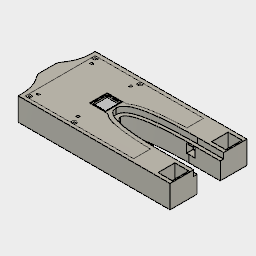
Plattan från fusion (Autodesk Fusion 360 design; units mm, degrees)
Autodesk Fusion 360 part; units mm, degrees
note: some values were not read from the file. Set by a fixed rule: which face or edge a step refers to.
(part 1 of 2)
sketch "Sketch1" plane through (0, 0, 0) normal (0, 1, 0) x (1, 0, 0)
  line L0 (220, -110) -> (0, -110)
  line L1 (0, -110) -> (0, 0)
  line L2 (220, -71.2097) -> (220, -110)
  line L3 (0, 0) -> (220, 0)
  line L4 (5, -5) -> (215, -5)
  line L5 (215, -5) -> (215, -33.4693)
  line L6 (180.0334, -33.4693) -> (215, -33.4693)
  spline S0 degree 3 poles (180.0334, -33.4693) (180.0317, -33.4693) (180.03, -33.4693) (180.0283, -33.4693) (159.0681, -33.512) (139.654, -34.3205) (124.0136, -36.2172) (115.4073, -37.2609) (107.9508, -38.6227) (101.8781, -40.4563) (97.9385, -41.6458) (94.574, -43.0141) (91.7704, -44.8227) (89.9877, -45.9727) (88.4083, -47.3156) (87.1811, -49.0361) (86.1319, -50.5071) (85.3713, -52.2924) (85.1516, -54.1891) (85.1143, -54.5109) (85.0919, -54.8348) (85.0844, -55.1587) (85.0841, -55.173) (85.0838, -55.1872) (85.0834, -55.2015) knots 0.561232 0.561232 0.561232 0.561232 0.561247 0.561247 0.561247 0.747063 0.747063 0.747063 0.849312 0.849312 0.849312 0.915644 0.915644 0.915644 0.957822 0.957822 0.957822 0.993882 0.993882 0.993882 1 1 1 1.000508 1.000508 1.000508 1.000508
  spline S1 degree 3 poles (85.0834, -55.2015) (85.0833, -55.2157) (85.0832, -55.23) (85.0832, -55.2442) (85.0717, -57.1054) (85.5912, -58.9664) (86.472, -60.5273) (87.5859, -62.5014) (89.1837, -64.0174) (90.9945, -65.2727) (93.6691, -67.1266) (96.8885, -68.4839) (100.6688, -69.6551) (106.9846, -71.6118) (114.9032, -72.9866) (124.1531, -73.9888) (139.7696, -75.6808) (159.1421, -76.258) (180.0619, -76.065) knots -0.00051 -0.00051 -0.00051 -0.00051 0 0 0 0.035213 0.035213 0.035213 0.079749 0.079749 0.079749 0.145527 0.145527 0.145527 0.255424 0.255424 0.255424 0.440962 0.440962 0.440962 0.440962
  line L7 (180.0619, -76.065) -> (215, -76.065)
  line L8 (215, -76.065) -> (215, -105)
  line L9 (215, -105) -> (5, -105)
  line L10 (5, -105) -> (5, -5)
  line L11 (220, -71.2097) -> (220, -76.065)
  line L12 (215, -92) -> (205, -92)
  line L13 (215, -18) -> (205, -18)
  circle A0 centre (205, -92) radius 2.7
  circle A1 centre (205, -18) radius 2.7
  circle A2 centre (205, -92) radius 5.25
  circle A3 centre (205, -18) radius 5.25
  line L14 (180.085, -81.065) -> (215, -81.065)
  spline S2 degree 3 poles (80.0838, -55.128) (80.0836, -55.1565) (80.0834, -55.1851) (80.0833, -55.2136) (80.0693, -57.4847) (80.5939, -59.807) (81.5103, -61.7976) (82.5316, -64.0162) (83.9716, -65.8142) (85.5066, -67.2576) (87.6935, -69.3141) (90.0877, -70.738) (92.6384, -71.9379) (96.4174, -73.7157) (100.6123, -74.9881) (105.3471, -76.0639) (113.1343, -77.8331) (122.3837, -79.0075) (132.8521, -79.8035) (146.8378, -80.8669) (162.9619, -81.2225) (180.085, -81.065) knots -0.00102 -0.00102 -0.00102 -0.00102 0 0 0 0.029213 0.029213 0.029213 0.061771 0.061771 0.061771 0.108156 0.108156 0.108156 0.176878 0.176878 0.176878 0.2899 0.2899 0.2899 0.440894 0.440894 0.440894 0.440894
  spline S3 degree 3 poles (180.0283, -28.4693) (180.0249, -28.4693) (180.0215, -28.4693) (180.0181, -28.4693) (162.2889, -28.5054) (145.6262, -29.0859) (131.2931, -30.4153) (122.4806, -31.2327) (114.5551, -32.326) (107.6808, -33.8168) (102.9997, -34.8321) (98.8082, -36.0189) (95.0386, -37.5637) (92.2561, -38.7039) (89.687, -40.0255) (87.3028, -41.8568) (85.5074, -43.2358) (83.7899, -44.9342) (82.4288, -47.164) (81.3112, -48.9949) (80.4774, -51.2077) (80.1955, -53.5241) (80.134, -54.0286) (80.0975, -54.5363) (80.0858, -55.0425) (80.0851, -55.071) (80.0844, -55.0995) (80.0838, -55.128) knots 0.561217 0.561217 0.561217 0.561217 0.561247 0.561247 0.561247 0.717499 0.717499 0.717499 0.813569 0.813569 0.813569 0.878987 0.878987 0.878987 0.927274 0.927274 0.927274 0.963637 0.963637 0.963637 0.993496 0.993496 0.993496 1 1 1 1.001016 1.001016 1.001016 1.001016
  line L15 (180.0283, -28.4693) -> (215, -28.4693)
  line L16 (205, -92) -> (195, -92)
  line L17 (195, -92) -> (195, -105)
  line L18 (195, -92) -> (195, -81.065)
  line L19 (195, -105) -> (160, -105)
  line L20 (160, -105) -> (160, -80.9937)
  line L21 (160, -28.7673) -> (160, -5)
  line L22 (160, -5) -> (195, -5)
  line L23 (195, -5) -> (195, -28.4693)
  line L24 (220, -33.4693) -> (220, -33.4693)
  line L25 (220, -76.065) -> (220.0001, -76.065)
  line L26 (160, -28.7673) -> (160, -33.7693)
  line L27 (195, -28.4693) -> (195, -33.4693)
  line L28 (195, -81.065) -> (195, -76.065)
  line L29 (160, -80.9937) -> (160, -75.9932)
  line L30 (215, -107.6) -> (2.4, -107.6)
  line L31 (2.4, -107.6) -> (2.4, -2.4)
  line L32 (2.4, -2.4) -> (215, -2.4)
  line L33 (215, -5) -> (215, -2.4)
  line L34 (215, -105) -> (215, -107.6)
  line L35 (80.0839, -55) -> (80.0868, -55)
  line L36 (80.0868, -55) -> (80.0868, -65)
  line L37 (80.0868, -65) -> (62.0868, -65)
  line L38 (62.0868, -65) -> (62.0868, -45)
  line L39 (62.0868, -45) -> (80.0868, -45)
  line L40 (80.0868, -45) -> (80.0868, -65)
  line L41 (82.0868, -67) -> (60.0868, -67)
  line L42 (60.0868, -67) -> (60.0868, -43)
  line L43 (60.0868, -43) -> (82.0868, -43)
  line L44 (82.0868, -43) -> (82.0868, -67)
  line L45 (80.8868, -65.8) -> (61.2868, -65.8)
  line L46 (61.2868, -65.8) -> (61.2868, -44.2)
  line L47 (61.2868, -44.2) -> (80.8868, -44.2)
  line L48 (80.8868, -44.2) -> (80.8868, -65.8)
  line L49 (215, -33.4693) -> (220, -33.4693)
  line L50 (215, -76.065) -> (220.0001, -76.065)
  spline S4 degree 3 poles (172.3167, -38.2821) (127.2999, -38.721) (91.6663, -43.1669) (91.3547, -54.7171) knots 0.588488 0.588488 0.588488 0.588488 1 1 1 1
  line L51 (172.3978, -71.2493) -> (220, -71.2097)
  line L52 (172.3167, -38.2821) -> (220, -38.2821)
  spline S5 degree 3 poles (91.3547, -54.7171) (91.1824, -66.3112) (127.02, -70.7779) (172.3978, -71.2493) knots 0 0 0 0 0.414646 0.414646 0.414646 0.414646
  line L53 (220, -76.065) -> (220, -71.2097)
  line L54 (220, -38.2821) -> (220, 0)
  line L55 (80.0868, -67.8) -> (59.2868, -67.8)
  line L56 (59.2868, -67.8) -> (59.2868, -42.2)
  line L57 (59.2868, -42.2) -> (80.0868, -42.2)
  line L58 (80.0868, -42.2) -> (86.8661, -42.2)
  line L59 (80.0868, -67.8) -> (86.1046, -67.8)
  dimension "d1" = 110
  dimension "d2" = 220
  dimension "d33" = 5.4
  dimension "d34" = 5.4
  dimension "d35" = 10.5
  dimension "d36" = 10.5
  dimension "d38" = 10
  dimension "d43" = 35
  dimension "d44" = 35
  dimension "d47" = 5
  dimension "d65" = 10
  dimension "d66" = 18
  dimension "d67" = 20
  dimension "d68" = 2
  dimension "d69" = 0.8
  dimension "d447" = 2.8
  measures "d1" distance of L1.end L0.end
  measures "d2" distance of L1.end L3.end
  measures "d33" diameter of A0
  measures "d34" diameter of A1
  measures "d35" diameter of A2
  measures "d36" diameter of A3
  measures "d38" distance of L12.end L16.end
  measures "d43" distance of L17.end L19.end
  measures "d44" distance of L21.end L22.end
  measures "d47" distance of L5.end L24.start
  measures "d65" distance of L35.end L36.end
  measures "d66" distance of L36.end L37.end
  measures "d67" distance of L36.end L39.end
extrude "Extrude51" add sketch "Sketch1" against normal blind 3 contours S2 S3 L41 L42 L43 L44 L55 L56 L57 L58 L59 | S2 S3 L41 L42 L43 L44 L45 L46 L47 L48 | S2 S3 L36 L37 L38 L39 L40 L45 L46 L47 L48 makes body 1
extrude "Extrude17" add sketch "Sketch1" along normal blind 0.7 separate body contours L0 L1 L2 L3 L5 L8 L30 L31 L32 L33 L34 L49 L50 L54 | L2 L6 S0 S1 L7 L11 L49 L50 S4 L51 L52 S5 L53 L54 | L7 L8 L14 L28 | S1 L7 L14 S2 L28 L29 | L9 L14 S2 L17 L18 L19 L20 | L5 L6 L15 L27 | S0 S1 S2 S3 L26 L29 L44 | L4 L9 L10 L19 L22 L30 L31 L32 L33 L34 | L6 S0 S3 L15 L26 L27 | L4 L9 L10 S2 S3 L20 L21 L55 L56 L57 L58 L59 | L4 S3 L15 L21 L22 L23 | S2 S3 L41 L42 L43 L44 L55 L56 L57 L58 L59 | S2 S3 L41 L42 L43 L44 L45 L46 L47 L48 | S2 S3 L44 L48 | S2 S3 L36 L37 L38 L39 L40 L45 L46 L47 L48 | S2 S3 L36 L40 L48 | S2 S3 L36 L37 L38 L39 L40 | S2 S3 L36 L40 makes body 2
extrude "Extrude15" add sketch "Sketch1" against normal blind 32 contours L0 L1 L2 L3 L5 L8 L30 L31 L32 L33 L34 L49 L50 L54 | L2 L6 S0 S1 L7 L11 L49 L50 S4 L51 L52 S5 L53 L54 bodies 2
extrude "Extrude18" add sketch "Sketch1" against normal blind 28 contours L7 L8 L14 L28 | S1 L7 L14 S2 L28 L29 | L9 L14 S2 L17 L18 L19 L20 | L5 L6 L15 L27 | S0 S1 S2 S3 L26 L29 L44 | L4 L9 L10 L19 L22 L30 L31 L32 L33 L34 | L6 S0 S3 L15 L26 L27 | L4 S3 L15 L21 L22 L23 | S2 S3 L44 L48 | S2 S3 L36 L40 L48 | S2 S3 L36 L40 bodies 2
extrude "Extrude19" cut sketch "Sketch1" along normal through all contours S2 S3 L36 L37 L38 L39 L40 bodies 2
sketch "Sketch7" plane through (0, 0, 0) normal (0, 0, -1) x (-1, 0, 0)
  line L0 (0, -32) -> (0, 0.7)
  line L1 (0, 0.7) -> (-220, 0.7)
  line L2 (-220, -32) -> (0, -32)
  line L3 (-220, 0.7) -> (-190, 0.7156)
  line L4 (-190, 0.7156) -> (-190, -32)
  line L5 (-181, -9.5928) -> (-180.9904, -9.5928)
  line L6 (-181, -9.5928) -> (-180.9904, -21.5928)
  line L7 (-180.9904, -21.5928) -> (-168.9904, -21.5928)
  line L8 (-168.9904, -21.5928) -> (-168.9904, -9.5928)
  line L9 (-168.9904, -9.5928) -> (-180.9904, -9.5928)
  line L10 (-180.9904, -9.5928) -> (-180.9904, -21.5928)
  line L11 (-190, -32) -> (-160, -32)
  line L12 (-160, -32) -> (-160, 0.7)
  line L13 (-220, 0.7) -> (-220, -32)
  dimension "d77" = 30
  dimension "d127" = 12
  dimension "d128" = 12
  dimension "d129" = 12
  dimension "d130" = 30
  measures "d77" distance of L1.end L3.end
  measures "d127" distance of L5.start L6.end
  measures "d128" distance of L6.end L5.end
  measures "d129" distance of L6.end L7.end
  measures "d130" distance of L4.end L11.end
extrude "Extrude25" cut sketch "Sketch7" against normal blind 10 from surface at -29 contours L7 L8 L9 L10 bodies 2
sketch "Sketch8" plane through (0, 0.7, 0) normal (0, 1, 0) x (-1, 0, 0)
  line L0 (-195, 105) -> (-195, 81.065)
  line L1 (-195, 81.065) -> (-215, 81.065)
  line L2 (-215, 81.065) -> (-215, 105)
  line L3 (-215, 105) -> (-195, 105)
  line L4 (-195, 5) -> (-215, 5)
  line L5 (-215, 5) -> (-215, 28.4693)
  line L6 (-215, 28.4693) -> (-195, 28.4693)
  line L7 (-195, 28.4693) -> (-195, 5)
  line L8 (-220, 0) -> (0, 0)
  line L9 (0, 0) -> (0, 110)
  line L10 (0, 110) -> (-220, 110)
  line L11 (-220, 110) -> (-220, 71.2097)
  line L12 (-220, 76.065) -> (-180.0619, 76.065)
  spline S0 degree 3 poles (-180.0619, 76.065) (-159.1795, 76.2576) (-139.8387, 75.6828) (-124.2368, 73.9979) (-115.6615, 73.0718) (-108.2229, 71.8213) (-102.1502, 70.0947) (-98.213, 68.9753) (-94.844, 67.6751) (-92.0221, 65.9426) (-90.1417, 64.7881) (-88.4752, 63.4272) (-87.1878, 61.6436) (-86.1381, 60.1892) (-85.3752, 58.4147) (-85.1541, 56.5302) (-85.104, 56.1036) (-85.0805, 55.6734) (-85.0832, 55.2442) (-85.0832, 55.23) (-85.0833, 55.2157) (-85.0834, 55.2015) knots -0.440962 -0.440962 -0.440962 -0.440962 -0.255755 -0.255755 -0.255755 -0.153959 -0.153959 -0.153959 -0.087961 -0.087961 -0.087961 -0.04398 -0.04398 -0.04398 -0.008119 -0.008119 -0.008119 0 0 0 0.00051 0.00051 0.00051 0.00051
  spline S1 degree 3 poles (-85.0834, 55.2015) (-85.0838, 55.1872) (-85.0841, 55.173) (-85.0844, 55.1587) (-85.1283, 53.2729) (-85.7115, 51.4171) (-86.6378, 49.8664) (-87.8395, 47.8546) (-89.5287, 46.3185) (-91.4514, 45.0322) (-94.4377, 43.0345) (-98.0815, 41.5688) (-102.3978, 40.3015) (-109.8672, 38.1085) (-119.3843, 36.5903) (-130.4817, 35.5147) (-144.8663, 34.1205) (-161.8701, 33.5063) (-180.0283, 33.4693) (-180.03, 33.4693) (-180.0317, 33.4693) (-180.0334, 33.4693) knots -1.000508 -1.000508 -1.000508 -1.000508 -1 -1 -1 -0.964386 -0.964386 -0.964386 -0.918178 -0.918178 -0.918178 -0.846413 -0.846413 -0.846413 -0.722224 -0.722224 -0.722224 -0.561247 -0.561247 -0.561247 -0.561232 -0.561232 -0.561232 -0.561232
  line L13 (-180.0334, 33.4693) -> (-220, 33.4693)
  line L14 (-172.3167, 38.2821) -> (-220, 38.2821)
  line L15 (-220, 38.2821) -> (-220, 0)
  line L16 (-220, 71.2097) -> (-172.3978, 71.2493)
  spline S2 degree 3 poles (-172.3978, 71.2493) (-127.02, 70.7779) (-91.1824, 66.3112) (-91.3547, 54.7171) knots -0.414646 -0.414646 -0.414646 -0.414646 0 0 0 0
  spline S3 degree 3 poles (-91.3547, 54.7171) (-91.6663, 43.1669) (-127.2999, 38.721) (-172.3167, 38.2821) knots -1 -1 -1 -1 -0.588488 -0.588488 -0.588488 -0.588488
  line L17 (-80.0868, 65) -> (-62.0868, 65)
  line L18 (-62.0868, 65) -> (-62.0868, 45)
  line L19 (-62.0868, 45) -> (-80.0868, 45)
  line L20 (-80.0868, 45) -> (-80.0868, 55)
  spline S4 degree 3 poles (-80.0868, 55) (-80.0864, 55.0142) (-80.0861, 55.0283) (-80.0858, 55.0425) (-80.0851, 55.071) (-80.0844, 55.0995) (-80.0838, 55.128) knots 0.999818 0.999818 0.999818 0.999818 1 1 1 1.001016 1.001016 1.001016 1.001016
  spline S5 degree 3 poles (-80.0838, 55.128) (-80.0836, 55.1565) (-80.0834, 55.1851) (-80.0833, 55.2136) (-80.0824, 55.354) (-80.0836, 55.4946) (-80.0868, 55.6354) knots -0.00102 -0.00102 -0.00102 -0.00102 0 0 0 0.001806 0.001806 0.001806 0.001806
  line L21 (-80.0868, 55.6354) -> (-80.0868, 65)
extrude "Extrude22" cut sketch "Sketch8" against normal blind 8 contours L11 L12 S0 S1 L13 L14 L15 L16 S2 S3 bodies 2
sketch "Sketch9" plane through (0, 0, 110) normal (0, 0, 1) x (1, 0, 0)
  line L0 (220, -32) -> (220, 0.7)
  line L1 (220, 0.7) -> (0, 0.7)
  line L2 (0, 0.7) -> (0, -32)
  line L3 (0, -32) -> (220, -32)
  line L4 (176.1, -28.0515) -> (176.1, -26.85)
  line L5 (173.9, -26.85) -> (173.9, -28.0515)
  arc A0 (176.1, -26.85) -> (173.9, -26.85) centre (175, -26.85) ccw
  line L6 (186.25, -16.7) -> (187.4515, -16.7)
  arc A1 (186.25, -14.5) -> (186.25, -16.7) centre (186.25, -15.6) ccw
  line L7 (187.4515, -14.5) -> (186.25, -14.5)
  line L8 (173.9, -3.1485) -> (173.9, -4.35)
  line L9 (176.1, -4.35) -> (176.1, -3.1485)
  arc A2 (173.9, -4.35) -> (176.1, -4.35) centre (175, -4.35) ccw
  line L10 (186.25, -16.7) -> (187.4515, -16.7)
  arc A3 (186.25, -14.5) -> (186.25, -16.7) centre (186.25, -15.6) ccw
  line L11 (173.9, -3.1485) -> (173.9, -4.35)
  line L12 (187.4515, -14.5) -> (186.25, -14.5)
  arc A4 (173.9, -4.35) -> (176.1, -4.35) centre (175, -4.35) ccw
  line L13 (158, -15.6) -> (158, -11.1)
  line L14 (176.1, -28.0515) -> (176.1, -26.85)
  line L15 (176.1, -4.35) -> (176.1, -3.1485)
  line L16 (173.9, -26.85) -> (173.9, -28.0515)
  arc A5 (176.1, -26.85) -> (173.9, -26.85) centre (175, -26.85) ccw
  arc A6 (176.1, -26.85) -> (173.9, -26.85) centre (175, -26.85) ccw
  arc A7 (173.9, -4.35) -> (176.1, -4.35) centre (175, -4.35) ccw
  line L17 (176.1, -4.35) -> (176.1, -3.1485)
  arc A8 (176.1, -26.85) -> (173.9, -26.85) centre (175, -26.85) ccw
  arc A9 (173.9, -4.35) -> (176.1, -4.35) centre (175, -4.35) ccw
  line L18 (176.1, -28.0515) -> (176.1, -26.85)
  line L19 (173.9, -26.85) -> (173.9, -28.0515)
  line L20 (186.25, -16.7) -> (187.4515, -16.7)
  line L21 (158, -15.6) -> (158, -20.1)
  line L22 (173.9, -3.1485) -> (173.9, -4.35)
  line L23 (176.1, -28.0515) -> (176.1, -26.85)
  line L24 (176.1, -4.35) -> (176.1, -3.1485)
  line L25 (173.9, -3.1485) -> (173.9, -4.35)
  line L26 (173.9, -26.85) -> (173.9, -28.0515)
  line L27 (187.4515, -14.5) -> (186.25, -14.5)
  arc A10 (186.25, -14.5) -> (186.25, -16.7) centre (186.25, -15.6) ccw
  line L28 (186.25, -16.7) -> (187.4515, -16.7)
  arc A11 (186.25, -14.5) -> (186.25, -16.7) centre (186.25, -15.6) ccw
  line L29 (187.4515, -14.5) -> (186.25, -14.5)
  arc A12 (173.9, -4.35) -> (176.1, -4.35) centre (175, -4.35) ccw
  arc A13 (173.9, -4.35) -> (176.1, -4.35) centre (175, -4.35) ccw
  arc A14 (173.9, -4.35) -> (176.1, -4.35) centre (175, -4.35) ccw
  arc A15 (173.9, -4.35) -> (176.1, -4.35) centre (175, -4.35) ccw
  line L30 (176.1, -4.35) -> (176.1, -3.1485)
  line L31 (173.9, -3.1485) -> (173.9, -4.35)
  line L32 (176.1, -4.35) -> (176.1, -3.1485)
  line L33 (173.9, -3.1485) -> (173.9, -4.35)
  line L34 (173.9, -3.1485) -> (173.9, -4.35)
  line L35 (176.1, -4.35) -> (176.1, -3.1485)
  line L36 (173.9, -3.1485) -> (173.9, -4.35)
  line L37 (158, -11.1) -> (164.3229, -9.1)
  line L38 (158, -20.1) -> (158, -30)
  arc A16 (176.1, -26.85) -> (173.9, -26.85) centre (175, -26.85) ccw
  line L39 (173.9, -26.85) -> (173.9, -28.0515)
  line L40 (186.25, -16.7) -> (187.4515, -16.7)
  line L41 (187.4515, -14.5) -> (186.25, -14.5)
  line L42 (187.4515, -14.5) -> (186.25, -14.5)
  line L43 (186.25, -16.7) -> (187.4515, -16.7)
  line L44 (187.4515, -14.5) -> (186.25, -14.5)
  arc A17 (186.25, -14.5) -> (186.25, -16.7) centre (186.25, -15.6) ccw
  arc A18 (186.25, -14.5) -> (186.25, -16.7) centre (186.25, -15.6) ccw
  line L45 (186.25, -16.7) -> (187.4515, -16.7)
  line L46 (187.4515, -14.5) -> (186.25, -14.5)
  line L47 (187.5, -15.6) -> (187.5, -30.0163)
  line L48 (173.9, -26.85) -> (173.9, -28.0515)
  line L49 (173.9, -26.85) -> (173.9, -28.0515)
  line L50 (173.9, -26.85) -> (173.9, -28.0515)
  arc A19 (176.1, -26.85) -> (173.9, -26.85) centre (175, -26.85) ccw
  arc A20 (186.25, -14.5) -> (186.25, -16.7) centre (186.25, -15.6) ccw
  arc A21 (186.25, -14.5) -> (186.25, -16.7) centre (186.25, -15.6) ccw
  line L51 (186.25, -16.7) -> (187.4515, -16.7)
  arc A22 (176.1, -26.85) -> (173.9, -26.85) centre (175, -26.85) ccw
  line L52 (176.1, -28.0515) -> (176.1, -26.85)
  arc A23 (176.1, -26.85) -> (173.9, -26.85) centre (175, -26.85) ccw
  line L53 (176.1, -28.0515) -> (176.1, -26.85)
  line L54 (176.1, -28.0515) -> (176.1, -26.85)
  line L55 (176.1, -28.0515) -> (176.1, -26.85)
  line L56 (176.1, -4.35) -> (176.1, -3.1485)
  arc A24 (173.9, -3.1485) -> (164.3229, -9.1) centre (175, -15.6) ccw
  arc A25 (173.9, -28.0515) -> (176.1, -28.0515) centre (175, -15.6) ccw
  arc A26 (173.9, -28.0515) -> (176.1, -28.0515) centre (175, -15.6) ccw
  arc A27 (187.4515, -16.7) -> (176.1, -3.1485) centre (175, -15.6) ccw
  arc A28 (173.9, -28.0515) -> (176.1, -28.0515) centre (175, -15.6) ccw
  arc A29 (173.9, -28.0515) -> (176.1, -28.0515) centre (175, -15.6) ccw
  arc A30 (173.9, -28.0515) -> (176.1, -28.0515) centre (175, -15.6) ccw
  arc A31 (173.9, -28.0515) -> (176.1, -28.0515) centre (175, -15.6) ccw
  arc A32 (187.4515, -16.7) -> (187.4515, -14.5) centre (175, -15.6) ccw
  line L57 (169, -9.6) -> (169, -21.6)
  line L58 (169, -21.6) -> (181, -21.6)
  line L59 (181, -21.6) -> (181, -9.6)
  line L60 (181, -9.6) -> (169, -9.6)
  line L61 (187.5, -30.0163) -> (158, -30)
  line L62 (176.1, -3.1485) -> (173.9, -3.1485)
  line L63 (158, -30, -110) -> (187.5, -30, -110)
  line L64 (176.1, -28.0515, -110) -> (176.1, -26.85, -110)
  line L65 (173.9, -26.85, -110) -> (173.9, -28.0515, -110)
  line L66 (176.1, -28.0515, -110) -> (176.1, -26.85, -110)
  line L67 (173.9, -26.85, -110) -> (173.9, -28.0515, -110)
  line L68 (176.1, -28.0515, -110) -> (176.1, -26.85, -110)
  arc A33 through (173.9, -28.0515, -110) (175, -28.1, -110) (176.1, -28.0515, -110)
  line L69 (176.1, -28.0515, -110) -> (176.1, -26.85, -110)
  arc A34 through (173.9, -28.0515, -110) (175, -28.1, -110) (176.1, -28.0515, -110)
  arc A35 through (173.9, -28.0515, -110) (175, -28.1, -110) (176.1, -28.0515, -110)
  arc A36 through (173.9, -28.0515, -110) (175, -28.1, -110) (176.1, -28.0515, -110)
  line L70 (187.5, -30.0163, -110) -> (158, -30, -110)
  arc A37 through (173.9, -28.0515, -110) (175, -28.1, -110) (176.1, -28.0515, -110)
  arc A38 through (173.9, -28.0515, -110) (175, -28.1, -110) (176.1, -28.0515, -110)
  line L71 (173.9, -26.85, -110) -> (173.9, -28.0515, -110)
  line L72 (186.25, -16.7, -110) -> (187.4515, -16.7, -110)
  line L73 (176.1, -4.35, -110) -> (176.1, -3.1485, -110)
  arc A39 through (176.1, -26.85, -110) (175, -25.75, -110) (173.9, -26.85, -110)
  arc A40 through (176.1, -26.85, -110) (175, -25.75, -110) (173.9, -26.85, -110)
  line L74 (176.1, -4.35, -110) -> (176.1, -3.1485, -110)
  arc A41 through (176.1, -26.85, -110) (175, -25.75, -110) (173.9, -26.85, -110)
  arc A42 through (186.25, -14.5, -110) (185.15, -15.6, -110) (186.25, -16.7, -110)
  arc A43 through (186.25, -14.5, -110) (185.15, -15.6, -110) (186.25, -16.7, -110)
  arc A44 through (186.25, -14.5, -110) (185.15, -15.6, -110) (186.25, -16.7, -110)
  line L75 (186.25, -16.7, -110) -> (187.4515, -16.7, -110)
  line L76 (173.9, -3.1485, -110) -> (173.9, -4.35, -110)
  arc A45 through (173.9, -4.35, -110) (175, -5.45, -110) (176.1, -4.35, -110)
  arc A46 through (173.9, -4.35, -110) (175, -5.45, -110) (176.1, -4.35, -110)
  line L77 (173.9, -26.85, -110) -> (173.9, -28.0515, -110)
  line L78 (187.4515, -14.5, -110) -> (186.25, -14.5, -110)
  line L79 (158, -15.6, -110) -> (158, -20.1, -110)
  arc A47 through (173.9, -4.35, -110) (175, -5.45, -110) (176.1, -4.35, -110)
  arc A48 through (173.9, -4.35, -110) (175, -5.45, -110) (176.1, -4.35, -110)
  arc A49 through (176.1, -26.85, -110) (175, -25.75, -110) (173.9, -26.85, -110)
  line L80 (173.9, -3.1485, -110) -> (173.9, -4.35, -110)
  line L81 (181, -21.6, -110) -> (181, -9.6, -110)
  arc A50 through (176.1, -26.85, -110) (175, -25.75, -110) (173.9, -26.85, -110)
  line L82 (173.9, -26.85, -110) -> (173.9, -28.0515, -110)
  line L83 (173.9, -3.1485, -110) -> (173.9, -4.35, -110)
  line L84 (187.5, -15.6, -110) -> (187.5, -30.0163, -110)
  line L85 (176.1, -3.1485, -110) -> (173.9, -3.1485, -110)
  line L86 (187.4515, -14.5, -110) -> (186.25, -14.5, -110)
  arc A51 through (176.1, -26.85, -110) (175, -25.75, -110) (173.9, -26.85, -110)
  line L87 (176.1, -4.35, -110) -> (176.1, -3.1485, -110)
  line L88 (176.1, -4.35, -110) -> (176.1, -3.1485, -110)
  arc A52 through (176.1, -26.85, -110) (175, -25.75, -110) (173.9, -26.85, -110)
  line L89 (176.1, -4.35, -110) -> (176.1, -3.1485, -110)
  line L90 (173.9, -3.1485, -110) -> (173.9, -4.35, -110)
  line L91 (169, -9.6, -110) -> (169, -21.6, -110)
  arc A53 through (173.9, -4.35, -110) (175, -5.45, -110) (176.1, -4.35, -110)
  line L92 (176.1, -4.35, -110) -> (176.1, -3.1485, -110)
  line L93 (187.4515, -14.5, -110) -> (186.25, -14.5, -110)
  line L94 (173.9, -26.85, -110) -> (173.9, -28.0515, -110)
  arc A54 through (173.9, -4.35, -110) (175, -5.45, -110) (176.1, -4.35, -110)
  line L95 (173.9, -3.1485, -110) -> (173.9, -4.35, -110)
  arc A55 through (187.4515, -16.7, -110) (187.5, -15.6, -110) (187.4515, -14.5, -110)
  line L96 (187.4515, -14.5, -110) -> (186.25, -14.5, -110)
  line L97 (158, -15.6, -110) -> (158, -11.1, -110)
  line L98 (158, -11.1, -110) -> (164.3229, -9.1, -110)
  arc A56 through (186.25, -14.5, -110) (185.15, -15.6, -110) (186.25, -16.7, -110)
  line L99 (173.9, -3.1485, -110) -> (173.9, -4.35, -110)
  line L100 (173.9, -26.85, -110) -> (173.9, -28.0515, -110)
  line L101 (176.1, -28.0515, -110) -> (176.1, -26.85, -110)
  line L102 (176.1, -28.0515, -110) -> (176.1, -26.85, -110)
  arc A57 through (173.9, -3.1485, -110) (168.4023, -4.983, -110) (164.3229, -9.1, -110)
  arc A58 through (186.25, -14.5, -110) (185.15, -15.6, -110) (186.25, -16.7, -110)
  line L103 (158, -20.1, -110) -> (158, -30, -110)
  arc A59 through (173.9, -4.35, -110) (175, -5.45, -110) (176.1, -4.35, -110)
  line L104 (181, -9.6, -110) -> (169, -9.6, -110)
  arc A60 through (173.9, -4.35, -110) (175, -5.45, -110) (176.1, -4.35, -110)
  line L105 (173.9, -26.85, -110) -> (173.9, -28.0515, -110)
  line L106 (176.1, -28.0515, -110) -> (176.1, -26.85, -110)
  line L107 (173.9, -3.1485, -110) -> (173.9, -4.35, -110)
  arc A61 through (176.1, -26.85, -110) (175, -25.75, -110) (173.9, -26.85, -110)
  arc A62 through (187.4515, -16.7, -110) (184.5824, -7.5733, -110) (176.1, -3.1485, -110)
  line L108 (176.1, -28.0515, -110) -> (176.1, -26.85, -110)
  line L109 (169, -21.6, -110) -> (181, -21.6, -110)
  line L110 (186.25, -16.7, -110) -> (187.4515, -16.7, -110)
  line L111 (186.25, -16.7, -110) -> (187.4515, -16.7, -110)
  line L112 (186.25, -16.7, -110) -> (187.4515, -16.7, -110)
  line L113 (187.4515, -14.5, -110) -> (186.25, -14.5, -110)
  line L114 (187.4515, -14.5, -110) -> (186.25, -14.5, -110)
  line L115 (186.25, -16.7, -110) -> (187.4515, -16.7, -110)
  line L116 (176.1, -4.35, -110) -> (176.1, -3.1485, -110)
  arc A63 through (186.25, -14.5, -110) (185.15, -15.6, -110) (186.25, -16.7, -110)
  line L117 (187.4515, -14.5, -110) -> (186.25, -14.5, -110)
  line L118 (187.4515, -14.5, -110) -> (186.25, -14.5, -110)
  line L119 (186.25, -16.7, -110) -> (187.4515, -16.7, -110)
  line L120 (186.25, -16.7, -110) -> (187.4515, -16.7, -110)
  arc A64 through (186.25, -14.5, -110) (185.15, -15.6, -110) (186.25, -16.7, -110)
  line L121 (176.1, -4.35, -110) -> (176.1, -3.1485, -110)
  line L122 (173.9, -3.1485, -110) -> (173.9, -4.35, -110)
  arc A65 through (186.25, -14.5, -110) (185.15, -15.6, -110) (186.25, -16.7, -110)
  dimension "d148" = 2.2
  dimension "d150" = 360
  dimension "d177" = 360
  dimension "d185" = 2.2
  dimension "d190" = 4.5
  dimension "d200" = 2.2
  dimension "d204" = 17
  dimension "d206" = 4.5
  dimension "d214" = 2.2
  dimension "d228" = 2.2
  dimension "d241" = 2.2
  dimension "d247" = 14.4163
  dimension "d252" = 25
  dimension "d254" = 2.2
  dimension "d267" = 2.2
  measures "d148" diameter of A0
  measures "d185" diameter of A5
  measures "d190" distance of L13.end L13.start
  measures "d200" diameter of A8
  measures "d204" distance of A24.centre L13.start
  measures "d206" distance of L21.end L13.start
  measures "d214" diameter of A6
  measures "d228" diameter of A23
  measures "d241" diameter of A22
  measures "d247" distance of L47.end L47.start
  measures "d252" diameter of A31
  measures "d254" diameter of A16
  measures "d267" diameter of A19
extrude "Extrude30" cut sketch "Sketch9" along normal blind 9 from surface at 20 contours L63 L72 L73 L74 A42 A43 A44 L75 L76 A45 A46 L78 L79 A47 A48 L80 L83 L84 L86 L87 L88 L89 L90 A53 L92 L93 A54 L95 A55 L96 L97 L98 A56 L99 A57 A58 L103 A59 A60 L107 A62 L110 L111 L112 L113 L114 L115 L116 A63 L117 L118 L119 L120 A64 L121 L122 A65 | L72 A42 A43 A44 L75 L78 L86 L93 A55 L96 A56 A58 A62 L110 L111 L112 L113 L114 L115 A63 L117 L118 L119 L120 A64 A65 | L73 L74 L76 A45 A46 A47 A48 L80 L83 L85 L87 L88 L89 L90 A53 L92 A54 L95 L99 A59 A60 L107 L116 L121 L122 | L64 L65 L66 L67 L68 A33 L69 A34 A35 A36 A37 A38 L71 A39 A40 A41 L77 A49 A50 L82 A51 A52 L94 L100 L101 L102 L105 L106 A61 L108 | L81 L91 L104 L109 in plane through (0, 0, 0) normal (0, 0, 1) bodies 2
extrude "Extrude31" cut sketch "Sketch9" against normal blind 9 from surface at -20 contours L4 L5 A0 L14 L16 A5 A6 A8 L18 L19 L23 L26 A16 L39 L48 L49 L50 A19 A22 L52 A23 L53 L54 L55 A25 A26 A28 A29 A30 A31 | L6 A1 L7 L10 A3 L12 L20 L27 A10 L28 A11 L29 L40 L41 L42 L43 L44 A17 A18 L45 L46 A20 A21 L51 A27 A32 | L6 A1 L7 L8 L9 A2 L10 A3 L11 L12 A4 L13 L15 A7 L17 A9 L20 L21 L22 L24 L25 L27 A10 L28 A11 L29 A12 A13 A14 A15 L30 L31 L32 L33 L34 L35 L36 L37 L38 L40 L41 L42 L43 L44 A17 A18 L45 L46 L47 A20 A21 L51 L56 A24 A27 A32 L61 | L8 L9 A2 L11 A4 L15 A7 L17 A9 L22 L24 L25 A12 A13 A14 A15 L30 L31 L32 L33 L34 L35 L36 L56 L62 | L57 L58 L59 L60 bodies 2
extrude "Extrude32" add sketch "Sketch9" against normal blind 1 from surface at -20 contours L4 L5 A0 L14 L16 A5 A6 A8 L18 L19 L23 L26 A16 L39 L48 L49 L50 A19 A22 L52 A23 L53 L54 L55 A25 A26 A28 A29 A30 A31 | L6 A1 L7 L10 A3 L12 L20 L27 A10 L28 A11 L29 L40 L41 L42 L43 L44 A17 A18 L45 L46 A20 A21 L51 A27 A32 | L8 L9 A2 L11 A4 L15 A7 L17 A9 L22 L24 L25 A12 A13 A14 A15 L30 L31 L32 L33 L34 L35 L36 L56 L62 bodies 2
extrude "Extrude33" add sketch "Sketch9" along normal blind 1 from surface at 20 contours L72 A42 A43 A44 L75 L78 L86 L93 A55 L96 A56 A58 A62 L110 L111 L112 L113 L114 L115 A63 L117 L118 L119 L120 A64 A65 | L73 L74 L76 A45 A46 A47 A48 L80 L83 L85 L87 L88 L89 L90 A53 L92 A54 L95 L99 A59 A60 L107 L116 L121 L122 | L64 L65 L66 L67 L68 A33 L69 A34 A35 A36 A37 A38 L71 A39 A40 A41 L77 A49 A50 L82 A51 A52 L94 L100 L101 L102 L105 L106 A61 L108 in plane through (0, 0, 0) normal (0, 0, 1) bodies 2
extrude "Extrude34" cut sketch "Sketch9" against normal blind 10 from surface at -29 contours L57 L58 L59 L60 bodies 2
sketch "Sketch12" plane through (0, 0, 0) normal (0, -1, 0) x (1, 0, 0)
  spline S0 degree 3 poles (80.0868, 55.6354) (80.1357, 57.7706) (80.6506, 59.9301) (81.5103, 61.7976) (82.5316, 64.0162) (83.9716, 65.8142) (85.5066, 67.2576) (87.6935, 69.3141) (90.0877, 70.738) (92.6384, 71.9379) (96.4174, 73.7157) (100.6123, 74.9881) (105.3471, 76.0639) (113.1343, 77.8331) (122.3837, 79.0075) (132.8521, 79.8035) (141.2176, 80.4396) (150.3482, 80.8224) (160, 80.9937) knots 0.001806 0.001806 0.001806 0.001806 0.029213 0.029213 0.029213 0.061771 0.061771 0.061771 0.108156 0.108156 0.108156 0.176878 0.176878 0.176878 0.2899 0.2899 0.2899 0.380217 0.380217 0.380217 0.380217
  line L0 (160, 80.9937) -> (160, 105)
  line L1 (160, 105) -> (5, 105)
  line L2 (5, 105) -> (5, 5)
  line L3 (5, 5) -> (160, 5)
  line L4 (160, 5) -> (160, 28.7673)
  spline S1 degree 3 poles (160, 28.7673) (149.7491, 29.0664) (140.083, 29.6001) (131.2931, 30.4153) (122.4806, 31.2327) (114.5551, 32.326) (107.6808, 33.8168) (102.9997, 34.8321) (98.8082, 36.0189) (95.0386, 37.5637) (92.2561, 38.7039) (89.687, 40.0255) (87.3028, 41.8568) (85.5074, 43.2358) (83.7899, 44.9342) (82.4288, 47.164) (81.3112, 48.9949) (80.4774, 51.2077) (80.1955, 53.5241) (80.1358, 54.0145) (80.0996, 54.5079) (80.0868, 55) knots 0.621676 0.621676 0.621676 0.621676 0.717499 0.717499 0.717499 0.813569 0.813569 0.813569 0.878987 0.878987 0.878987 0.927274 0.927274 0.927274 0.963637 0.963637 0.963637 0.993496 0.993496 0.993496 0.999818 0.999818 0.999818 0.999818
  circle A0 centre (8, 102) radius 3
  line L5 (72, 99) -> (72, 11)
  line L6 (8, 11) -> (8, 99)
  circle A1 centre (8, 8) radius 3
  circle A2 centre (72, 8) radius 3
  circle A3 centre (72, 102) radius 3
  line L7 (69, 8) -> (11, 8)
  line L8 (11, 102) -> (69, 102)
  circle A4 centre (72, 102) radius 1.25
  circle A5 centre (72, 8) radius 1.25
  circle A6 centre (8, 8) radius 1.25
  circle A7 centre (8, 102) radius 1.25
  line L9 (10, 95) -> (70, 95)
  line L10 (70, 95) -> (70, 15)
  line L11 (70, 15) -> (10, 15)
  line L12 (10, 15) -> (10, 95)
  line L13 (10, 95) -> (12, 95)
  line L14 (12, 95) -> (12, 93)
  line L15 (12, 93) -> (10, 93)
  line L16 (10, 93) -> (10, 95)
  circle A8 centre (12, 93) radius 2
  circle A9 centre (12, 93) radius 1.25
  line L17 (70, 95) -> (68, 95)
  line L18 (68, 95) -> (68, 94.3274)
  line L19 (68, 94.3274) -> (68, 92.3274)
  circle A10 centre (68, 92.3274) radius 2
  circle A11 centre (68, 92.3274) radius 1.25
  line L20 (70, 15) -> (68, 15)
  line L21 (68, 15) -> (68, 17)
  line L22 (68, 17) -> (70, 17)
  line L23 (70, 17) -> (70, 15)
  circle A12 centre (68, 17) radius 2
  circle A13 centre (68, 17) radius 1.25
  line L24 (10, 15) -> (12, 15)
  line L25 (12, 15) -> (12, 17)
  line L26 (12, 17) -> (10, 17)
  line L27 (10, 17) -> (10, 15)
  circle A14 centre (12, 17) radius 2
  circle A15 centre (12, 17) radius 1.25
  line L28 (80.0868, 55) -> (80.0868, 45)
  line L29 (80.0868, 45) -> (62.0868, 45)
  line L30 (62.0868, 45) -> (62.0868, 65)
  line L31 (62.0868, 65) -> (80.0868, 65)
  line L32 (80.0868, 65) -> (80.0868, 55.6354)
  dimension "d317" = 6
  dimension "d319" = 94
  dimension "d320" = 64
  dimension "d321" = 6
  dimension "d323" = 6
  dimension "d325" = 6
  dimension "d378" = 2.5
  dimension "d379" = 2.5
  dimension "d380" = 2.5
  dimension "d381" = 2.5
  dimension "d396" = 60
  dimension "d397" = 80
  dimension "d398" = 2
  dimension "d399" = 2
  dimension "d400" = 4
  dimension "d401" = 2.5
  dimension "d402" = 2
  dimension "d403" = 2
  dimension "d404" = 2.5
  dimension "d405" = 2
  dimension "d406" = 2
  dimension "d407" = 2.5
  dimension "d408" = 2
  dimension "d409" = 2
  dimension "d410" = 2.5
  measures "d317" diameter of A0
  measures "d319" distance of A0.centre A1.centre
  measures "d320" distance of A0.centre A3.centre
  measures "d321" diameter of A1
  measures "d323" diameter of A2
  measures "d325" diameter of A3
  measures "d378" diameter of A4
  measures "d379" diameter of A5
  measures "d380" diameter of A6
  measures "d381" diameter of A7
  measures "d396" distance of L9.start L9.end
  measures "d397" distance of L9.start L11.end
  measures "d398" distance of L9.start L15.end
  measures "d399" distance of L9.start L13.end
  measures "d400" diameter of A8
  measures "d401" diameter of A9
  measures "d402" distance of L9.end L17.end
  measures "d403" distance of L18.end L19.end
  measures "d404" diameter of A11
  measures "d405" distance of L10.end L20.end
  measures "d406" distance of L10.end L22.end
  measures "d407" diameter of A13
  measures "d408" distance of L11.end L24.end
  measures "d409" distance of L11.end L26.end
  measures "d410" diameter of A15
extrude "Extrude44" add sketch "Sketch12" along normal blind 5 contours A10 | L21 L22 A12 A13 | L21 L22 A12 A13 | L25 L26 A14 A15 | L25 L26 A14 A15 | L14 L15 A8 A9 | L14 L15 A8 A9 bodies 2
extrude "Extrude35" add sketch "Sketch12" along normal blind 12 contours A3 | A0 | A2 | A1 bodies 2
sketch "Sketch13" plane through (0, -28, 0) normal (0, -1, 0) x (1, 0, 0)
  line L0 (187.5, 81) -> (160, 81)
  line L1 (160, 81) -> (160, 80.9937)
  spline S0 degree 3 poles (160, 80.9937) (150.3482, 80.8224) (141.2176, 80.4396) (132.8521, 79.8035) (122.3837, 79.0075) (113.1343, 77.8331) (105.3471, 76.0639) (100.6123, 74.9881) (96.4174, 73.7157) (92.6384, 71.9379) (90.0877, 70.738) (87.6935, 69.3141) (85.5066, 67.2576) (83.9716, 65.8142) (82.5316, 64.0162) (81.5103, 61.7976) (80.5939, 59.807) (80.0693, 57.4847) (80.0833, 55.2136) (80.0834, 55.1851) (80.0836, 55.1565) (80.0838, 55.128) knots -0.380217 -0.380217 -0.380217 -0.380217 -0.2899 -0.2899 -0.2899 -0.176878 -0.176878 -0.176878 -0.108156 -0.108156 -0.108156 -0.061771 -0.061771 -0.061771 -0.029213 -0.029213 -0.029213 0 0 0 0.00102 0.00102 0.00102 0.00102
  spline S1 degree 3 poles (80.0838, 55.128) (80.0844, 55.0995) (80.0851, 55.071) (80.0858, 55.0425) (80.0975, 54.5363) (80.134, 54.0286) (80.1955, 53.5241) (80.4774, 51.2077) (81.3112, 48.9949) (82.4288, 47.164) (83.7899, 44.9342) (85.5074, 43.2358) (87.3028, 41.8568) (89.687, 40.0255) (92.2561, 38.7039) (95.0386, 37.5637) (98.8082, 36.0189) (102.9997, 34.8321) (107.6808, 33.8168) (114.5551, 32.326) (122.4806, 31.2327) (131.2931, 30.4153) (139.5092, 29.6533) (148.4908, 29.1373) (158, 28.8289) knots -1.001016 -1.001016 -1.001016 -1.001016 -1 -1 -1 -0.993496 -0.993496 -0.993496 -0.963637 -0.963637 -0.963637 -0.927274 -0.927274 -0.927274 -0.878987 -0.878987 -0.878987 -0.813569 -0.813569 -0.813569 -0.717499 -0.717499 -0.717499 -0.627932 -0.627932 -0.627932 -0.627932
  line L2 (158, 28.8289) -> (158, 29)
  line L3 (158, 29) -> (187.5, 29)
  line L4 (187.5, 29) -> (187.5, 20)
  line L5 (187.5, 20) -> (176.1, 20)
  line L6 (176.1, 20) -> (173.9, 20)
  line L7 (173.9, 20) -> (160, 20)
  line L8 (160, 20) -> (160, 5)
  line L9 (160, 5) -> (5, 5)
  line L10 (5, 5) -> (5, 105)
  line L11 (5, 105) -> (160, 105)
  line L12 (160, 105) -> (160, 90)
  line L13 (160, 90) -> (173.9, 90)
  line L14 (173.9, 90) -> (176.1, 90)
  line L15 (176.1, 90) -> (187.5, 90)
  line L16 (187.5, 90) -> (187.5, 81)
  line L17 (195, 81.065) -> (195, 105)
  line L18 (195, 105) -> (215, 105)
  line L19 (215, 105) -> (215, 107.6)
  line L20 (215, 107.6) -> (2.4, 107.6)
  line L21 (2.4, 107.6) -> (2.4, 2.4)
  line L22 (2.4, 2.4) -> (215, 2.4)
  line L23 (215, 2.4) -> (215, 5)
  line L24 (215, 5) -> (195, 5)
  line L25 (195, 5) -> (195, 28.4693)
  line L26 (195, 28.4693) -> (215, 28.4693)
  line L27 (215, 28.4693) -> (215, 33.4693)
  line L28 (215, 33.4693) -> (180.0334, 33.4693)
  spline S2 degree 3 poles (85.0834, 55.2015) (85.1068, 54.1955) (85.2621, 52.759) (86.4016, 50.2112) (87.0737, 48.9777) (89.9279, 45.9257) (92.1317, 44.3816) (100.5133, 40.4492) (107.8482, 38.6647) (136.8603, 33.9502) (164.5729, 33.5008) (180.0334, 33.4693) knots -9.827045 -9.827045 -9.827045 -9.827045 -8.213218 -8.213218 -7.416849 -7.416849 -6.408432 -6.408432 -4.638162 -4.638162 0 0 0 0
  spline S3 degree 3 poles (180.0619, 76.065) (166.0703, 76.1941) (150.913, 75.9958) (122.4781, 74.134) (110.7492, 72.5443) (96.8266, 68.5789) (93.9137, 67.0804) (90.5259, 65.0507) (89.1724, 63.956) (86.8287, 61.3733) (86.2047, 60.0899) (85.0703, 57.3337) (85.0806, 55.657) (85.0834, 55.2015) knots -0.389228 -0.389228 -0.389228 -0.389228 -0.329659 -0.329659 -0.267908 -0.267908 -0.229652 -0.229652 -0.187711 -0.187711 -0.136677 -0.136677 0 0 0 0
  line L29 (180.0619, 76.065) -> (215, 76.065)
  line L30 (215, 76.065) -> (215, 81.065)
  line L31 (215, 81.065) -> (195, 81.065)
  line L32 (215, 33.4693) -> (190, 33.4693)
  line L33 (190, 33.4693) -> (190.0609, 2.4)
  line L34 (215, 2.4) -> (190.0609, 2.4)
  line L35 (215, 2.4) -> (215, 33.4693)
  line L36 (215, 107.6) -> (190, 107.6)
  line L37 (190, 107.6) -> (215, 107.6)
  line L38 (215, 107.6) -> (215, 76.065)
  line L39 (215, 76.065) -> (190, 76.065)
  line L40 (190, 76.065) -> (190, 107.6)
  dimension "d329" = 25
  dimension "d330" = 25
  measures "d329" distance of L27.end L32.end
  measures "d330" distance of L19.end L36.end
extrude "Extrude36" add sketch "Sketch13" against normal blind 4 from surface at 4 contours L17 L18 L19 L20 L29 L30 L31 L36 L37 L38 L39 L40 | L17 L18 L31 L38 | L22 L23 L24 L25 L26 L27 L28 L32 L33 L34 L35 | L24 L25 L26 L35 bodies 2
extrude "Extrude37" cut sketch "Sketch1" against normal through all contours L12 A0 L16 | L12 A0 L16 | A1 bodies 2
sketch "Sketch15" plane through (0, 0, 105) normal (0, 0, -1) x (-1, 0, 0)
  line L0 (-72, 0) -> (-160, 0)
  line L1 (-160, 0) -> (-160, -28)
  line L2 (-160, -28) -> (-5, -28)
  line L3 (-5, -28) -> (-5, 0)
  line L4 (-5, 0) -> (-8, 0)
  line L5 (-8, 0) -> (-72, 0)
  line L6 (-5, -28) -> (-5, -23)
  line L7 (-8, 0) -> (-8, -12)
  line L8 (-8, -12) -> (-8, 0)
  line L9 (-72, 0) -> (-72, -12)
  line L10 (-72, -12) -> (-72, 0)
  dimension "d342" = 5
  measures "d342" distance of L2.end L6.end
sketch "Sketch16" plane through (0, -28, 0) normal (0, -1, 0) x (1, 0, 0)
  line L0 (187.5, 81) -> (160, 81)
  line L1 (160, 81) -> (160, 80.9937)
  spline S0 degree 3 poles (160, 80.9937) (150.3482, 80.8224) (141.2176, 80.4396) (132.8521, 79.8035) (122.3837, 79.0075) (113.1343, 77.8331) (105.3471, 76.0639) (100.6123, 74.9881) (96.4174, 73.7157) (92.6384, 71.9379) (90.0877, 70.738) (87.6935, 69.3141) (85.5066, 67.2576) (83.9716, 65.8142) (82.5316, 64.0162) (81.5103, 61.7976) (80.5939, 59.807) (80.0693, 57.4847) (80.0833, 55.2136) (80.0834, 55.1851) (80.0836, 55.1565) (80.0838, 55.128) knots -0.380217 -0.380217 -0.380217 -0.380217 -0.2899 -0.2899 -0.2899 -0.176878 -0.176878 -0.176878 -0.108156 -0.108156 -0.108156 -0.061771 -0.061771 -0.061771 -0.029213 -0.029213 -0.029213 0 0 0 0.00102 0.00102 0.00102 0.00102
  spline S1 degree 3 poles (80.0838, 55.128) (80.0844, 55.0995) (80.0851, 55.071) (80.0858, 55.0425) (80.0975, 54.5363) (80.134, 54.0286) (80.1955, 53.5241) (80.4774, 51.2077) (81.3112, 48.9949) (82.4288, 47.164) (83.7899, 44.9342) (85.5074, 43.2358) (87.3028, 41.8568) (89.687, 40.0255) (92.2561, 38.7039) (95.0386, 37.5637) (98.8082, 36.0189) (102.9997, 34.8321) (107.6808, 33.8168) (114.5551, 32.326) (122.4806, 31.2327) (131.2931, 30.4153) (139.5092, 29.6533) (148.4908, 29.1373) (158, 28.8289) knots -1.001016 -1.001016 -1.001016 -1.001016 -1 -1 -1 -0.993496 -0.993496 -0.993496 -0.963637 -0.963637 -0.963637 -0.927274 -0.927274 -0.927274 -0.878987 -0.878987 -0.878987 -0.813569 -0.813569 -0.813569 -0.717499 -0.717499 -0.717499 -0.627932 -0.627932 -0.627932 -0.627932
  line L2 (158, 28.8289) -> (158, 29)
  line L3 (158, 29) -> (187.5, 29)
  line L4 (187.5, 29) -> (187.5, 20)
  line L5 (187.5, 20) -> (176.1, 20)
  line L6 (176.1, 20) -> (173.9, 20)
  line L7 (173.9, 20) -> (160, 20)
  line L8 (160, 20) -> (160, 5)
  line L9 (160, 5) -> (5, 5)
  line L10 (5, 5) -> (5, 105)
  line L11 (5, 105) -> (160, 105)
  line L12 (160, 105) -> (160, 90)
  line L13 (160, 90) -> (173.9, 90)
  line L14 (173.9, 90) -> (176.1, 90)
  line L15 (176.1, 90) -> (187.5, 90)
  line L16 (187.5, 90) -> (187.5, 81)
  line L17 (190.0609, 2.4) -> (190, 33.4693)
  line L18 (190, 33.4693) -> (180.0334, 33.4693)
  spline S2 degree 3 poles (85.0834, 55.2015) (85.1068, 54.1955) (85.2621, 52.759) (86.4016, 50.2112) (87.0737, 48.9777) (89.9279, 45.9257) (92.1317, 44.3816) (100.5133, 40.4492) (107.8482, 38.6647) (136.8603, 33.9502) (164.5729, 33.5008) (180.0334, 33.4693) knots -9.827045 -9.827045 -9.827045 -9.827045 -8.213218 -8.213218 -7.416849 -7.416849 -6.408432 -6.408432 -4.638162 -4.638162 0 0 0 0
  spline S3 degree 3 poles (180.0619, 76.065) (166.0703, 76.1941) (150.913, 75.9958) (122.4781, 74.134) (110.7492, 72.5443) (96.8266, 68.5789) (93.9137, 67.0804) (90.5259, 65.0507) (89.1724, 63.956) (86.8287, 61.3733) (86.2047, 60.0899) (85.0703, 57.3337) (85.0806, 55.657) (85.0834, 55.2015) knots -0.389228 -0.389228 -0.389228 -0.389228 -0.329659 -0.329659 -0.267908 -0.267908 -0.229652 -0.229652 -0.187711 -0.187711 -0.136677 -0.136677 0 0 0 0
  line L19 (180.0619, 76.065) -> (190, 76.065)
  line L20 (190, 76.065) -> (190, 107.6)
  line L21 (190, 107.6) -> (2.4, 107.6)
  line L22 (2.4, 107.6) -> (2.4, 2.4)
  line L23 (2.4, 2.4) -> (190.0609, 2.4)
  line L24 (5, 105) -> (10, 105)
  line L25 (10, 105) -> (10, 100)
  line L26 (10, 100) -> (5, 100)
  line L27 (5, 100) -> (5, 105)
  dimension "d343" = 5
  dimension "d344" = 5
  measures "d343" distance of L10.end L24.end
  measures "d344" distance of L10.end L26.end
sketch "Sketch17" plane through (0, 0, 105) normal (0, 0, -1) x (-1, 0, 0)
  line L0 (-72, 0) -> (-160, 0)
  line L1 (-160, 0) -> (-160, -28)
  line L2 (-160, -28) -> (-5, -28)
  line L3 (-5, -28) -> (-5, 0)
  line L4 (-5, 0) -> (-8, 0)
  line L5 (-8, 0) -> (-72, 0)
  line L6 (-5, -28) -> (-5, -18)
  line L7 (-8, 0) -> (-8, -12)
  line L8 (-8, -12) -> (-8, 0)
  line L9 (-72, 0) -> (-72, -12)
  line L10 (-72, -12) -> (-72, 0)
  dimension "d345" = 10
  measures "d345" distance of L2.end L6.end
sketch "Sketch18" plane through (0, -28, 0) normal (0, -1, 0) x (1, 0, 0)
  line L0 (187.5, 81) -> (160, 81)
  line L1 (160, 81) -> (160, 80.9937)
  spline S0 degree 3 poles (160, 80.9937) (150.3482, 80.8224) (141.2176, 80.4396) (132.8521, 79.8035) (122.3837, 79.0075) (113.1343, 77.8331) (105.3471, 76.0639) (100.6123, 74.9881) (96.4174, 73.7157) (92.6384, 71.9379) (90.0877, 70.738) (87.6935, 69.3141) (85.5066, 67.2576) (83.9716, 65.8142) (82.5316, 64.0162) (81.5103, 61.7976) (80.5939, 59.807) (80.0693, 57.4847) (80.0833, 55.2136) (80.0834, 55.1851) (80.0836, 55.1565) (80.0838, 55.128) knots -0.380217 -0.380217 -0.380217 -0.380217 -0.2899 -0.2899 -0.2899 -0.176878 -0.176878 -0.176878 -0.108156 -0.108156 -0.108156 -0.061771 -0.061771 -0.061771 -0.029213 -0.029213 -0.029213 0 0 0 0.00102 0.00102 0.00102 0.00102
  spline S1 degree 3 poles (80.0838, 55.128) (80.0844, 55.0995) (80.0851, 55.071) (80.0858, 55.0425) (80.0975, 54.5363) (80.134, 54.0286) (80.1955, 53.5241) (80.4774, 51.2077) (81.3112, 48.9949) (82.4288, 47.164) (83.7899, 44.9342) (85.5074, 43.2358) (87.3028, 41.8568) (89.687, 40.0255) (92.2561, 38.7039) (95.0386, 37.5637) (98.8082, 36.0189) (102.9997, 34.8321) (107.6808, 33.8168) (114.5551, 32.326) (122.4806, 31.2327) (131.2931, 30.4153) (139.5092, 29.6533) (148.4908, 29.1373) (158, 28.8289) knots -1.001016 -1.001016 -1.001016 -1.001016 -1 -1 -1 -0.993496 -0.993496 -0.993496 -0.963637 -0.963637 -0.963637 -0.927274 -0.927274 -0.927274 -0.878987 -0.878987 -0.878987 -0.813569 -0.813569 -0.813569 -0.717499 -0.717499 -0.717499 -0.627932 -0.627932 -0.627932 -0.627932
  line L2 (158, 28.8289) -> (158, 29)
  line L3 (158, 29) -> (187.5, 29)
  line L4 (187.5, 29) -> (187.5, 20)
  line L5 (187.5, 20) -> (176.1, 20)
  line L6 (176.1, 20) -> (173.9, 20)
  line L7 (173.9, 20) -> (160, 20)
  line L8 (160, 20) -> (160, 5)
  line L9 (160, 5) -> (5, 5)
  line L10 (5, 5) -> (5, 105)
  line L11 (5, 105) -> (160, 105)
  line L12 (160, 105) -> (160, 90)
  line L13 (160, 90) -> (173.9, 90)
  line L14 (173.9, 90) -> (176.1, 90)
  line L15 (176.1, 90) -> (187.5, 90)
  line L16 (187.5, 90) -> (187.5, 81)
  line L17 (190.0609, 2.4) -> (190, 33.4693)
  line L18 (190, 33.4693) -> (180.0334, 33.4693)
  spline S2 degree 3 poles (85.0834, 55.2015) (85.1068, 54.1955) (85.2621, 52.759) (86.4016, 50.2112) (87.0737, 48.9777) (89.9279, 45.9257) (92.1317, 44.3816) (100.5133, 40.4492) (107.8482, 38.6647) (136.8603, 33.9502) (164.5729, 33.5008) (180.0334, 33.4693) knots -9.827045 -9.827045 -9.827045 -9.827045 -8.213218 -8.213218 -7.416849 -7.416849 -6.408432 -6.408432 -4.638162 -4.638162 0 0 0 0
  spline S3 degree 3 poles (180.0619, 76.065) (166.0703, 76.1941) (150.913, 75.9958) (122.4781, 74.134) (110.7492, 72.5443) (96.8266, 68.5789) (93.9137, 67.0804) (90.5259, 65.0507) (89.1724, 63.956) (86.8287, 61.3733) (86.2047, 60.0899) (85.0703, 57.3337) (85.0806, 55.657) (85.0834, 55.2015) knots -0.389228 -0.389228 -0.389228 -0.389228 -0.329659 -0.329659 -0.267908 -0.267908 -0.229652 -0.229652 -0.187711 -0.187711 -0.136677 -0.136677 0 0 0 0
  line L19 (180.0619, 76.065) -> (190, 76.065)
  line L20 (190, 76.065) -> (190, 107.6)
  line L21 (190, 107.6) -> (2.4, 107.6)
  line L22 (2.4, 107.6) -> (2.4, 2.4)
  line L23 (2.4, 2.4) -> (190.0609, 2.4)
  line L24 (5, 105) -> (12.5, 105)
  line L25 (12.5, 105) -> (12.5, 97.5)
  line L26 (12.5, 97.5) -> (5, 97.5)
  line L27 (5, 97.5) -> (5, 105)
  line L28 (5, 5) -> (12.5, 5)
  line L29 (12.5, 5) -> (12.5, 12.5)
  line L30 (12.5, 12.5) -> (5, 12.5)
  line L31 (5, 12.5) -> (5, 5)
  dimension "d348" = 7.5
  dimension "d349" = 7.5
  dimension "d356" = 7.5
  dimension "d357" = 7.5
  measures "d348" distance of L10.end L24.end
  measures "d349" distance of L10.end L26.end
  measures "d356" distance of L9.end L28.end
  measures "d357" distance of L9.end L30.end